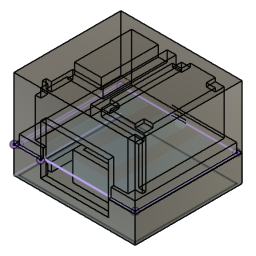
Astrobot clock v14 (Autodesk Fusion 360 design; units mm, degrees)
Autodesk Fusion 360 part; units mm, degrees
note: some values were not read from the file. Set by a fixed rule: which face or edge a step refers to.
sketch "Sketch1" plane through (0, 0, 0) normal (0, 0, 1) x (1, 0, 0)
  line L0 (0, 0) -> (62, 0)
  line L1 (62, 0) -> (62, 60)
  line L2 (62, 60) -> (0, 60)
  line L3 (0, 60) -> (0, 0)
  dimension "d1" = 62
  dimension "d2" = 60
  constraint horizontal L0
  constraint vertical L1
  constraint horizontal L2
  constraint vertical L3
  constraint coincident L0.start L3.end
  measures "d1" distance of L0.start L0.end
  measures "d2" distance of L0.start L2.end
extrude "Extrude2" add sketch "Sketch1" along normal blind 50 makes body 1
shell "Shell1" thickness 3 removed faces 0 bodies 1
sketch "Sketch2" plane through (0, 0, 0) normal (0, -1, 0) x (1, 0, 0)
  line L0 (0, 0) -> (62, 0)
  line L1 (62, 0) -> (62, 50)
  line L2 (62, 50) -> (0, 50)
  line L3 (0, 50) -> (0, 0)
  line L4 (9, 34) -> (47, 34)
  line L5 (47, 34) -> (47, 6)
  line L6 (47, 6) -> (9, 6)
  line L7 (9, 6) -> (9, 34)
  dimension "d8" = 38
  dimension "d9" = 28
  constraint horizontal L4
  constraint vertical L5
  constraint horizontal L6
  constraint vertical L7
  measures "d8" distance of L4.start L4.end
  measures "d9" distance of L4.start L6.end
extrude "Extrude3" cut sketch "Sketch2" against normal blind 4 contours L4 L5 L6 L7 bodies 1
sketch "Sketch3" plane through (59, 0, 0) normal (-1, 0, 0) x (0, -1, 0)
  line L0 (-57, 3) -> (-3, 3)
  line L1 (-3, 3) -> (-3, 47)
  line L2 (-3, 47) -> (-57, 47)
  line L3 (-57, 47) -> (-57, 3)
  line L4 (-3, 47) -> (-7, 47)
  line L5 (-7, 47) -> (-7, 3)
  line L6 (-7, 3) -> (-3, 3)
  line L7 (-3, 3) -> (-3, 47)
  line L8 (-9, 47) -> (-57, 47)
  line L9 (-57, 47) -> (-57, 3)
  line L10 (-57, 3) -> (-9, 3)
  line L11 (-9, 3) -> (-9, 47)
  constraint horizontal L4
  constraint vertical L5
  constraint horizontal L6
  constraint vertical L7
  constraint coincident L1.end L2.start
  constraint horizontal L8
  constraint vertical L9
  constraint horizontal L10
  constraint vertical L11
  constraint coincident L0.start L3.end
  constraint coincident L2 L8.start
extrude "Extrude4" add sketch "Sketch3" along normal blind 4 contours L0 L2 L3 L8 L9 L10 L11 | L0 L1 L2 L4 L5 L6 L7 bodies 1
sketch "Sketch4" plane through (3, 0, 0) normal (1, 0, 0) x (0, 1, 0)
  line L0 (3, 3) -> (57, 3)
  line L1 (57, 3) -> (57, 47)
  line L2 (57, 47) -> (3, 47)
  line L3 (3, 47) -> (3, 3)
  line L4 (3, 47) -> (7, 47)
  line L5 (7, 47) -> (7, 42)
  line L6 (7, 42) -> (3, 42)
  line L7 (3, 42) -> (3, 47)
  line L8 (3, 3) -> (7, 3)
  line L9 (7, 3) -> (7, 8)
  line L10 (7, 8) -> (3, 8)
  line L11 (3, 8) -> (3, 3)
  line L12 (9, 47) -> (57, 47)
  line L13 (57, 47) -> (57, 42)
  line L14 (57, 42) -> (9, 42)
  line L15 (9, 42) -> (9, 47)
  line L16 (9, 3) -> (57, 3)
  line L17 (57, 3) -> (57, 8)
  line L18 (57, 8) -> (9, 8)
  line L19 (9, 8) -> (9, 3)
  constraint horizontal L4
  constraint vertical L5
  constraint horizontal L6
  constraint vertical L7
  constraint coincident L2.end L3.start
  constraint horizontal L8
  constraint vertical L9
  constraint horizontal L10
  constraint vertical L11
  constraint coincident L0.start L3.end
  constraint horizontal L12
  constraint vertical L13
  constraint horizontal L14
  constraint vertical L15
  constraint coincident L2 L12.start
  constraint horizontal L16
  constraint vertical L17
  constraint horizontal L18
  constraint vertical L19
  constraint coincident L1 L17.end
  constraint coincident L0 L16.start
  constraint coincident L1 L13.end
extrude "Extrude5" add sketch "Sketch4" along normal blind 3 contours L0 L3 L8 L9 L10 L11 | L0 L1 L16 L17 L18 L19 | L2 L3 L4 L5 L6 L7 | L1 L2 L12 L13 L14 L15 bodies 1
extrude "Extrude19" add 1 faces at (0, 40, 33.3333) along direction (-1, 0, 0) blind 6 on bodies 1 bodies 1
ref_plane "WorkPlane1" through (0, 0, 15) normal (0, 0, 1) x (1, 0, 0)
split "Split1" by plane through (0, 0, 15) normal (0, 0, 1) bodies 1 makes body 2 at (39.3333, 40, 50)
sketch "Sketch7" plane through (0, 0, 0) normal (0, 0, -1) x (1, 0, 0)
  line L0 (-6, -60) -> (62, -60)
  line L1 (62, -60) -> (62, 0)
  line L2 (62, 0) -> (-6, 0)
  line L3 (-6, 0) -> (-6, -60)
  line L4 (60.5, -1.5) -> (-4.5, -1.5)
  line L5 (-4.5, -1.5) -> (-4.5, -58.5)
  line L6 (-4.5, -58.5) -> (60.5, -58.5)
  line L7 (60.5, -58.5) -> (60.5, -1.5)
  dimension "d18" = -1.5
sketch "Sketch8" plane through (0, 0, 15) normal (0, 0, 1) x (-1, 0, 0)
  line L0 (-62, -60) -> (6, -60)
  line L1 (-47, 0) -> (-62, 0)
  line L2 (-9, 0) -> (-9, -3)
  line L3 (-9, -3) -> (-3, -3)
  line L4 (-3, -3) -> (-3, -57)
  line L5 (-3, -57) -> (-55, -57)
  line L6 (-55, -57) -> (-55, -9)
  line L7 (-55, -9) -> (-59, -9)
  line L8 (-59, -9) -> (-59, -7)
  line L9 (-59, -7) -> (-55, -7)
  line L10 (-55, -7) -> (-55, -3)
  line L11 (-55, -3) -> (-47, -3)
  line L12 (-47, -3) -> (-47, 0)
  line L13 (-62, 0) -> (-62, -60)
  line L14 (4.5, -58.5) -> (-60.5, -58.5)
  line L15 (-60.5, -1.5) -> (4.5, -1.5)
  line L16 (-60.5, -58.5) -> (-60.5, -1.5)
  line L17 (6, -60) -> (6, 0)
  line L18 (6, 0) -> (-9, 0)
  line L19 (-60.5, -58.5) -> (-60.5, -1.5)
  line L20 (-60.5, -1.5) -> (4.5, -1.5)
  line L21 (4.5, -58.5) -> (-60.5, -58.5)
  line L22 (4.5, -1.5) -> (4.5, -58.5)
extrude "Extrude6" add sketch "Sketch8" along normal blind 5 contours L2 L3 L4 L5 L6 L7 L8 L9 L10 L11 L12 L14 L15 L16 L19 L20 L21 L22 bodies 1
combine "Combine1" operation cut target body 2 tool bodies 1 keep tools
sketch "Sketch9" plane through (0, 0, 47) normal (0, 0, -1) x (1, 0, 0)
  line L0 (6, -9) -> (6, -57)
  line L1 (6, -57) -> (55, -57)
  line L2 (55, -57) -> (55, -9)
  line L3 (55, -9) -> (59, -9)
  line L4 (59, -9) -> (59, -7)
  line L5 (59, -7) -> (55, -7)
  line L6 (55, -7) -> (55, -3)
  line L7 (55, -3) -> (6, -3)
  line L8 (6, -3) -> (6, -7)
  line L9 (6, -7) -> (3, -7)
  line L10 (3, -7) -> (3, -9)
  line L11 (3, -9) -> (6, -9)
  line L12 (3, -57) -> (18, -57)
  line L13 (18, -57) -> (18, -25)
  line L14 (18, -25) -> (3, -25)
  line L15 (3, -25) -> (3, -57)
  line L16 (3, -57) -> (23, -57)
  line L17 (23, -57) -> (23, -21)
  line L18 (23, -21) -> (3, -21)
  line L19 (3, -21) -> (3, -57)
  dimension "d21" = 15
  dimension "d22" = 32
  dimension "d23" = 20
  dimension "d24" = 36
  constraint horizontal L12
  constraint vertical L13
  constraint horizontal L14
  constraint vertical L15
  constraint horizontal L16
  constraint vertical L17
  constraint horizontal L18
  constraint vertical L19
  measures "d21" distance of L12.start L12.end
  measures "d22" distance of L12.start L14.end
  measures "d23" distance of L12.start L16.end
  measures "d24" distance of L12.start L18.end
extrude "Extrude7" add sketch "Sketch9" along normal blind 5 contours L0 L1 L12 L13 L14 L16 bodies 2
extrude "Extrude8" add sketch "Sketch9" along normal blind 6 contours L0 L1 L13 L14 L16 L17 L18 | L0 L14 L18 L19 bodies 2
extrude "Extrude9" cut 2 faces at (4, 46.3333, 42) (10, 46.3333, 42) along direction (0, 0, 1) blind 5 on bodies 2 bodies 2
sketch "Sketch10" plane through (0, 0, 47) normal (0, 0, -1) x (1, 0, 0)
  line L0 (55, -57) -> (31, -57)
  line L1 (31, -57) -> (31, -12)
  line L2 (31, -12) -> (55, -12)
  line L3 (55, -12) -> (55, -57)
  line L4 (55, -57) -> (28, -57)
  line L5 (28, -57) -> (28, -9)
  line L6 (28, -9) -> (55, -9)
  line L7 (55, -9) -> (55, -57)
  line L8 (55, -57) -> (50, -57)
  line L9 (50, -57) -> (50, -52)
  line L10 (50, -52) -> (55, -52)
  line L11 (55, -52) -> (55, -57)
  line L12 (55, -12) -> (50, -12)
  line L13 (50, -12) -> (50, -17)
  line L14 (50, -17) -> (55, -17)
  line L15 (55, -17) -> (55, -12)
  line L16 (31, -12) -> (36, -12)
  line L17 (36, -12) -> (36, -17)
  line L18 (36, -17) -> (31, -17)
  line L19 (31, -17) -> (31, -12)
  line L20 (31, -57) -> (36, -57)
  line L21 (36, -57) -> (36, -52)
  line L22 (36, -52) -> (31, -52)
  line L23 (31, -52) -> (31, -57)
  dimension "d31" = 24
  dimension "d32" = 45
  dimension "d33" = 27
  dimension "d34" = 48
  dimension "d37" = 5
  dimension "d38" = 5
  dimension "d39" = 5
  dimension "d40" = 5
  dimension "d41" = 5
  dimension "d42" = 5
  dimension "d43" = 5
  dimension "d44" = 5
  constraint horizontal L0
  constraint vertical L1
  constraint horizontal L2
  constraint vertical L3
  constraint horizontal L4
  constraint vertical L5
  constraint horizontal L6
  constraint vertical L7
  constraint horizontal L8
  constraint vertical L9
  constraint horizontal L10
  constraint vertical L11
  constraint horizontal L12
  constraint vertical L13
  constraint horizontal L14
  constraint vertical L15
  constraint horizontal L16
  constraint vertical L17
  constraint horizontal L18
  constraint vertical L19
  constraint horizontal L20
  constraint vertical L21
  constraint horizontal L22
  constraint vertical L23
  measures "d31" distance of L0.start L0.end
  measures "d32" distance of L0.start L2.end
  measures "d33" distance of L0.start L4.end
  measures "d34" distance of L0.start L6.end
  measures "d37" distance of L0.start L8.end
  measures "d38" distance of L0.start L10.end
  measures "d39" distance of L2.end L12.end
  measures "d40" distance of L2.end L14.end
  measures "d41" distance of L1.end L16.end
  measures "d42" distance of L1.end L18.end
  measures "d43" distance of L0.end L20.end
  measures "d44" distance of L0.end L22.end
extrude "Extrude10" add sketch "Sketch10" along normal blind 6 contours L1 L2 L4 L5 L6 L7 L12 L16 L19 L23 bodies 2
extrude "Extrude11" add sketch "Sketch10" along normal blind 2 contours L0 L3 L4 L7 L8 L9 L10 L11 | L0 L1 L4 L20 L21 L22 L23 | L2 L3 L7 L12 L13 L14 L15 | L1 L2 L16 L17 L18 L19 bodies 2
sketch "Sketch12" plane through (0, 0, 3) normal (0, 0, 1) x (-1, 0, 0)
  line L0 (-6, -9) -> (-3, -9)
  line L1 (-3, -9) -> (-3, -7)
  line L2 (-3, -7) -> (-6, -7)
  line L3 (-6, -7) -> (-6, -3)
  line L4 (-6, -3) -> (-55, -3)
  line L5 (-55, -3) -> (-55, -7)
  line L6 (-55, -7) -> (-59, -7)
  line L7 (-59, -7) -> (-59, -9)
  line L8 (-59, -9) -> (-55, -9)
  line L9 (-55, -9) -> (-55, -57)
  line L10 (-55, -57) -> (-6, -57)
  line L11 (-6, -57) -> (-6, -9)
  line L12 (-20, -57) -> (-38, -57)
  line L13 (-38, -57) -> (-38, -13)
  line L14 (-38, -13) -> (-20, -13)
  line L15 (-20, -13) -> (-20, -57)
  line L16 (-20, -57) -> (-17, -57)
  line L17 (-17, -57) -> (-17, -13)
  line L18 (-17, -13) -> (-20, -13)
  line L19 (-20, -13) -> (-20, -57)
  line L20 (-38, -57) -> (-41, -57)
  line L21 (-41, -57) -> (-41, -13)
  line L22 (-41, -13) -> (-38, -13)
  line L23 (-38, -13) -> (-38, -57)
  line L24 (-17, -13) -> (-41, -13)
  line L25 (-41, -13) -> (-41, -10)
  line L26 (-41, -10) -> (-17, -10)
  line L27 (-17, -10) -> (-17, -13)
  dimension "d49" = 18
  dimension "d50" = 44
  dimension "d51" = 3
  dimension "d52" = 44
  dimension "d53" = 3
  dimension "d54" = 44
  dimension "d55" = 24
  dimension "d56" = 3
  constraint horizontal L12
  constraint vertical L13
  constraint horizontal L14
  constraint vertical L15
  constraint coincident L10 L12.start
  constraint horizontal L16
  constraint vertical L17
  constraint horizontal L18
  constraint vertical L19
  constraint horizontal L20
  constraint vertical L21
  constraint horizontal L22
  constraint vertical L23
  constraint horizontal L24
  constraint vertical L25
  constraint horizontal L26
  constraint vertical L27
  measures "d49" distance of L12.start L12.end
  measures "d50" distance of L12.start L14.end
  measures "d51" distance of L12.start L16.end
  measures "d52" distance of L12.start L14.end
  measures "d53" distance of L12.end L20.end
  measures "d54" distance of L12.end L13.end
  measures "d55" distance of L17.end L21.end
  measures "d56" distance of L17.end L26.end
extrude "Extrude12" add sketch "Sketch12" along normal blind 16 contours L10 L15 L16 L17 L18 L19 L24 | L14 L18 L22 L24 L25 L26 L27 | L10 L13 L20 L21 L22 L23 L24 bodies 1
extrude "Extrude13" add 1 faces at (26, 42.3333, 3) along direction (0, 0, 1) blind 1 on bodies 1 bodies 1
sketch "Sketch13" plane through (0, 0, 4) normal (0, 0, 1) x (-1, 0, 0)
  line L0 (-38, -13) -> (-38, -57)
  line L1 (-38, -57) -> (-20, -57)
  line L2 (-20, -57) -> (-20, -13)
  line L3 (-20, -13) -> (-38, -13)
  line L4 (-20, -57) -> (-22, -57)
  line L5 (-22, -57) -> (-22, -55)
  line L6 (-22, -55) -> (-20, -55)
  line L7 (-20, -55) -> (-20, -57)
  line L8 (-38, -57) -> (-36, -57)
  line L9 (-36, -57) -> (-36, -55)
  line L10 (-36, -55) -> (-38, -55)
  line L11 (-38, -55) -> (-38, -57)
  line L12 (-20, -13) -> (-22, -13)
  line L13 (-22, -13) -> (-22, -15)
  line L14 (-22, -15) -> (-20, -15)
  line L15 (-20, -15) -> (-20, -13)
  line L16 (-38, -13) -> (-36, -13)
  line L17 (-36, -13) -> (-36, -15)
  line L18 (-36, -15) -> (-38, -15)
  line L19 (-38, -15) -> (-38, -13)
  dimension "d61" = 2
  dimension "d62" = 2
  dimension "d63" = 2
  dimension "d64" = 2
  dimension "d65" = 2
  dimension "d66" = 2
  dimension "d67" = 2
  dimension "d68" = 2
  constraint horizontal L4
  constraint vertical L5
  constraint horizontal L6
  constraint vertical L7
  constraint coincident L1.end L2.start
  constraint horizontal L8
  constraint vertical L9
  constraint horizontal L10
  constraint vertical L11
  constraint coincident L0.end L1.start
  constraint horizontal L12
  constraint vertical L13
  constraint horizontal L14
  constraint vertical L15
  constraint coincident L2.end L3.start
  constraint horizontal L16
  constraint vertical L17
  constraint horizontal L18
  constraint vertical L19
  constraint coincident L0.start L3.end
  measures "d61" distance of L1.end L4.end
  measures "d62" distance of L1.end L6.end
  measures "d63" distance of L0.end L8.end
  measures "d64" distance of L0.end L10.end
  measures "d65" distance of L2.end L12.end
  measures "d66" distance of L2.end L14.end
  measures "d67" distance of L0.start L16.end
  measures "d68" distance of L0.start L18.end
extrude "Extrude14" add sketch "Sketch13" along normal blind 10 contours L0 L3 L16 L17 L18 L19 | L0 L1 L8 L9 L10 L11 | L2 L3 L12 L13 L14 L15 | L1 L2 L4 L5 L6 L7 bodies 1
sketch "Sketch14" plane through (0, 57, 0) normal (0, -1, 0) x (1, 0, 0)
  line L0 (55, 20) -> (3, 20)
  line L1 (22, 14) -> (36, 14)
  line L2 (24, 14) -> (34, 14)
  line L3 (34, 14) -> (34, 9)
  line L4 (34, 9) -> (24, 9)
  line L5 (24, 9) -> (24, 14)
  line L6 (22, 14) -> (22, 4)
  line L7 (22, 4) -> (36, 4)
  line L8 (36, 4) -> (36, 14)
  line L9 (20, 14) -> (22, 14)
  line L10 (36, 14) -> (38, 14)
  line L11 (38, 14) -> (38, 19)
  line L12 (20, 19) -> (20, 14)
  line L13 (38, 19) -> (41, 19)
  line L14 (41, 19) -> (41, 3)
  line L15 (41, 3) -> (55, 3)
  line L16 (55, 3) -> (55, 20)
  line L17 (3, 20) -> (3, 8)
  line L18 (3, 8) -> (6, 8)
  line L19 (6, 8) -> (6, 3)
  line L20 (6, 3) -> (17, 3)
  line L21 (17, 3) -> (17, 19)
  line L22 (17, 19) -> (20, 19)
  dimension "d71" = 10
  dimension "d72" = 5
  constraint horizontal L2
  constraint vertical L3
  constraint horizontal L4
  constraint vertical L5
  constraint coincident L1 L2.start
  constraint coincident L1.end L8.end
  constraint coincident L1.start L6.start
  measures "d71" distance of L2.start L2.end
  measures "d72" distance of L2.start L4.end
extrude "Extrude17" cut sketch "Sketch14" against normal blind 5 contours L1 L2 L3 L4 L5 bodies 1
extrude "Extrude18" cut 1 faces at (27.3333, 58, 14) along direction (0, 0, 1) blind 11 on bodies 1 bodies 1
named bodies: "bottom", "top"
